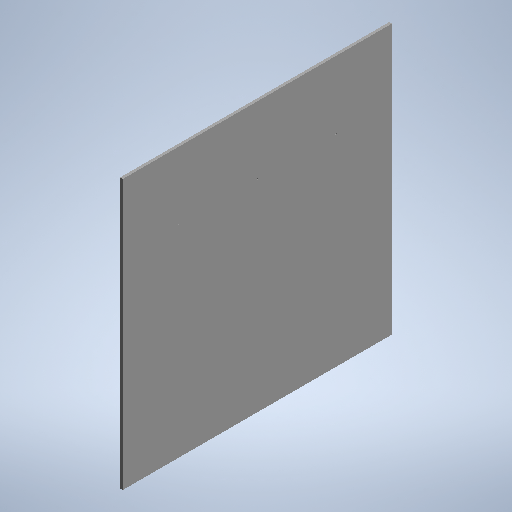
# Autodesk Inventor part: RT_FRM_MC_009_ElectricalBackPlate
Saved by Autodesk Inventor 2025.4 (Build 294407000, 407)
## iProperties
Created: 2026-05-16
Part Number: RT_FRM_MC_009_ElectricalBackPlate
Material: Générique
Document SubType Name: Modeling
Designer: louis
Density: 1 g/cm^3
Appearance: Par défaut
Author: louis
Autodesk Inventor part; units mm, degrees
ref_plane "YZ Plane" through (0, 0, 0) normal (1, 0, 0) x (0, 1, 0)
ref_plane "XZ Plane" through (0, 0, 0) normal (0, 1, 0) x (-1, 0, 0)
ref_plane "XY Plane" through (0, 0, 0) normal (0, 0, 1) x (1, 0, 0)
sketch "Sketch2" plane through (0, 0, 0) normal (1, 0, 0) x (0, 1, 0)
  line L0 (-300, -300) -> (300, -300)
  line L1 (300, -300) -> (300, 300)
  line L2 (300, 300) -> (-300, 300)
  line L3 (-300, 300) -> (-300, -300)
  line L4 (-300, -300) -> (300, 300) construction
  line L5 (300, -300) -> (-300, 300) construction
  point P0 (0, 0)
  dimension "d0" = 600
  dimension "d1" = 600
  constraints: 12 end point, 2 midpoint, 2 parallel, 1 horizontal, 1 perpendicular
  measures "d0" distance of L2.end L1.end
  measures "d1" distance of L1.end L0.end
extrude "Extrusion1" add sketch "Sketch2" along normal blind 6
sketch "Sketch3" plane through (6, 0, 0) normal (1, 0, 0) x (0, 0, -1)
  line L0 (-150, -175) -> (-150, 175) construction
  line L1 (0, 0) -> (-150, 0) construction
  dimension "d4" = 350
  dimension "d5" = 150
  constraints: 4 end point, 3 coincident, 1 horizontal, 1 midpoint, 1 vertical
  measures "d4" distance of L0.start L0.end
  measures "d5" distance of L1.start L1.end
hole "Hole1" at (6, -175, 150) at (6, 175, 150) at (6, 0, 150) direction (-1, 0, 0) diameter 3 end through all
body "Solid1"
